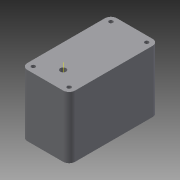
# Autodesk Inventor part: herkulex
Saved by Autodesk Inventor 2015 (Build 190159000, 159)
## iProperties
Created: 2014-10-18
Part Number: herkulex
Material: Generic
Document SubType Name: Modeling
Designer: ericd_000
Density: 1 g/cm^3
Appearance: Default
Author: ericd_000
Autodesk Inventor part; units mm, degrees
ref_plane "YZ Plane" through (0, 0, 0) normal (1, 0, 0) x (0, 1, 0)
ref_plane "XZ Plane" through (0, 0, 0) normal (0, 1, 0) x (-1, 0, 0)
ref_plane "XY Plane" through (0, 0, 0) normal (0, 0, 1) x (1, 0, 0)
sketch "Sketch1" plane through (0, 0, 0) normal (0, 0, 1) x (1, 0, 0)
  line L0 (-12, 22.5) -> (12, 22.5)
  line L1 (12, 22.5) -> (12, -22.5)
  line L2 (12, -22.5) -> (-12, -22.5)
  line L3 (-12, -22.5) -> (-12, 22.5)
  point P0 (0, 0)
  point P1 (12, 0)
  point P2 (0, 22.5)
  dimension "d0" = 24
  dimension "d1" = 45
  constraints: 8 end point, 2 midpoint, 2 parallel, 1 horizontal, 1 horizontal alignment, 1 perpendicular, 1 vertical alignment
  measures "d0" distance of L0.start L0.end
  measures "d1" distance of L2.end L0.start
extrude "Extrusion1" add sketch "Sketch1" along normal blind 31
fillet "Fillet1" radius 3 4 edges at (12, 22.5, 15.5) (-12, 22.5, 15.5) (12, -22.5, 15.5) (-12, -22.5, 15.5)
sketch "Sketch3" plane through (0, 0, 31) normal (0, 0, 1) x (1, 0, 0)
  line L0 (0, -22.5) -> (0, -13.5) construction
  circle A0 centre (0, -13.5) radius 1.5
  point P0 (0, 0)
  dimension "d8" = 9
  dimension "d9" = 3
  constraints: 2 end point, 1 centre point, 1 coincident, 1 vertical
  measures "d8" distance of L0.start L0.end
  measures "d9" diameter of A0
extrude "Extrusion3" cut sketch "Sketch3" against normal blind 5
sketch "Sketch4" plane through (0, 0, 31) normal (0, 0, 1) x (1, 0, 0)
  circle A0 centre (-9, 19.5) radius 1
  circle A1 centre (9, 19.5) radius 1
  circle A2 centre (-9, -19.5) radius 1
  circle A3 centre (9, -19.5) radius 1
  line L0 (-12, 19.5) -> (-12, -19.5) projected
  line L1 (9, 22.5) -> (-9, 22.5) projected
  line L2 (12, -19.5) -> (12, 19.5) projected
  line L3 (-9, -22.5) -> (9, -22.5) projected
  point P0 (0, 0)
  dimension "d12" = 2
  dimension "d13" = 3
  dimension "d14" = 3
  dimension "d15" = 3
  dimension "d16" = 3
  dimension "d17" = 3
  dimension "d18" = 3
  dimension "d19" = 3
  dimension "d20" = 3
  dimension "d21" = 2
  dimension "d22" = 2
  dimension "d23" = 2
  constraints: 4 centre point
  measures "d12" diameter of A2
  measures "d13" distance from line of A0.centre L0
  measures "d14" distance from line of L1 A0.centre
  measures "d15" distance from line of A1.centre L1
  measures "d16" distance from line of A1.centre L2
  measures "d17" distance from line of A2.centre L0
  measures "d18" distance from line of A2.centre L3
  measures "d19" distance from line of A3.centre L3
  measures "d20" distance from line of A3.centre L2
  measures "d21" diameter of A0
  measures "d22" diameter of A1
  measures "d23" diameter of A3
extrude "Extrusion4" cut sketch "Sketch4" against normal up to surface (31 mm away)
body "Solid1"
